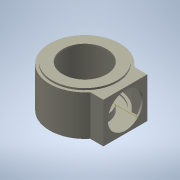
# Autodesk Inventor part: Robot-Axis5
Saved by Autodesk Inventor 2021 (Build 250183000, 183)
## iProperties
Created: 2001-08-22
Part Number: Robot-Axis5
Document SubType Name: ﾓﾃﾞﾘﾝｸﾞ
Designer: Administrator
Density: 1 g/cm^3
Material: Generic
Appearance: Smooth - Ivory
Control State: 0
Master: False
Checked Out: False
Shininess: 21.0
Length Units: 11269
Angle Units: 11279
Time Units: 11290
Mass Units: 11283
Length Display Precision: 3
Angle Display Precision: 2
Density: 0.0
Volumn: 0.0
Area: 0.0
PropertySet Name: Model Information
Author: Administrator
Autodesk Inventor part; units mm, degrees
ref_plane "YZ Plane" through (0, 0, 0) normal (1, 0, 0) x (0, 1, 0)
ref_plane "XZ Plane" through (0, 0, 0) normal (0, 1, 0) x (-1, 0, 0)
sketch "ｽｹｯﾁ1" plane through (0, 0, 0) normal (0, 0, 1) x (1, 0, 0)
  circle A0 centre (0, 0) radius 40
  dimension "d0" = 80
  constraints: 1 centre point
  measures "d0" diameter of A0
extrude "押し出し1" add sketch "ｽｹｯﾁ1" along normal mid plane 40
sketch "ｽｹｯﾁ2" plane through (0, 0, 20) normal (0, 0, 1) x (1, 0, 0)
  circle A0 centre (0, 0) radius 40 projected
  circle A1 centre (0, 0) radius 37
  dimension "d3" = 3
  constraints: 1 centre point
  measures "d3" radial gap between concentric circles of A0 A1
extrude "押し出し2" add sketch "ｽｹｯﾁ2" along normal blind 2 contours A1
mirror "Mirror1" about plane through (0, 0, 0) normal (0, 0, 1) of "押し出し2"
ref_plane "作業平面1" through (0, 0, 0) normal (1, 0, 0) x (0, 1, 0)
sketch "ｽｹｯﾁ3" plane through (0, 0, 0) normal (1, 0, 0) x (0, 1, 0)
  line L0 (-37, -22) -> (37, -22) projected
  line L1 (40, -20) -> (-40, -20) projected
  line L2 (-25, 26) -> (25, 26)
  line L3 (25, 26) -> (25, -20)
  line L4 (25, -20) -> (-25, -20)
  line L5 (-25, -20) -> (-25, 26)
  line L6 (-25, 3) -> (25, 3)
  line L7 (0, 26) -> (0, -20)
  line L8 (0, -20) -> (0, 24.715)
  dimension "d6" = 50
  dimension "d7" = 46
  dimension "d8" = 25
  constraints: 14 end point, 6 midpoint, 2 collinear, 2 parallel, 2 perpendicular, 1 horizontal, 1 point on line
  measures "d6" distance of L2.start L2.end
  measures "d7" distance of L4.end L2.start
  measures "d8" distance between parallel lines of L5 L7
extrude "押し出し3" add sketch "ｽｹｯﾁ3" along normal blind 46.2
sketch "Sketch4" plane through (46.2, 0, 0) normal (1, 0, 0) x (0, 0, -1)
  point P0 (0, 0)
ref_plane "Work Plane2" through (46.2, 0, -20) normal (0, -1, 0) x (1, 0, 0)
ref_plane "Work Plane3" through (46.2, 25, 3) normal (0, 0, -1) x (-1, 0, 0)
shell "Shell1" thickness 2 removed faces 0
sketch "Sketch7" plane through (0, 0, 22) normal (0, 0, 1) x (1, 0, 0)
  circle A0 centre (0, 0) radius 37 projected
hole "Hole1" at (0, 0, 22) direction (0, 0, -1) diameter 50 end through all
sketch "Sketch8" plane through (46.2, 0, 0) normal (1, 0, 0) x (0, 0, -1)
  point P0 (-3, 0)
hole "Hole2" at (46.2, 0, 3) direction (-1, 0, 0) diameter 40 depth 2 tip angle 118
sketch "Sketch9" plane through (0, 0, -22) normal (0, 0, -1) x (-1, 0, 0)
  circle A0 centre (0, 0) radius 25
  constraints: 1 centre point, 1 coincident
extrude "Extrusion7" add sketch "Sketch9" against normal blind 10
sketch "Sketch10" plane through (0, 0, -22) normal (0, 0, -1) x (-1, 0, 0)
  circle A0 centre (0, 0) radius 25 projected
  circle A1 centre (0, 0) radius 25
  constraints: 1 centre point, 1 coincident
extrude "Extrusion8" cut sketch "Sketch10" against normal blind 10
body "Solid1"
